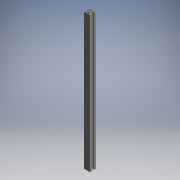
# Autodesk Inventor part: NFSF5-2020-437-Z6-YA10-YB427
Saved by Autodesk Inventor 2017.3 (Build 213256000, 256)
## iProperties
Part Number: NFSF5-2020-437-Z6-YA10-YB427
Material: Generic
Catalog Web Link: www.cadenas.de
Description: NFS5-2020, NFSB5-2020, HFS5-2020, HFSB5-2020, CAF5-2020, HFSY5-2020, NFSF5-2020, HFSF5-2020, HFSFB5-2020, NFST5-2020, HFST5-2020, HFSTB5-2020, HFSH5-2020, HFSC5-2020-HFS5 Series Aluminum Extrusions 20 Square -1 Slot-
Vendor: MISUMI
Document SubType Name: Modeling
Designer: partserver
Manufacturer: MISUMI
Mass: 84.1199 g
Surface Area: 795.09 cm^2
Volume: 84.1199 cm^3
Density: 1 g/cm^3
Appearance: PSOLRGB-175-175-175
Category: PARTsolutions
Company: MISUMI
Title: NFSF5-2020-437-Z6-YA10-YB427
Author: Cadenas PARTsolutions
Comments: HFS5 Series Aluminum Extrusions 20 Square -1 Slot-
PSOL_IDENT_0: {$CADENAS_DATA\23d-libs\misumi\metric\38_al_extrusions_blackets\5\hfs5_2020.prj},706 {VTYP=3D},{NB=N
PSOL_IDENT_1: FSF5-2020-437-Z6-YA10-YB427},{LINA=NFSF5-2020-437-Z6-YA10-YB427},{NN=NFS5-2020, NFSB5-2020, HFS5-202
PSOL_IDENT_2: 0, HFSB5-2020, CAF5-2020, HFSY5-2020, NFSF5-2020, HFSF5-2020, HFSFB5-2020, NFST5-2020, HFST5-2020, H
PSOL_IDENT_3: FSTB5-2020, HFSH5-2020, HFSC5-2020},{DATE=09.09.2019 15:28:27},{GEOMDATE=18.06.2019 07:59:14},{VERSI
PSOL_IDENT_4: ON=},{LINEID=40},{WBVAR=L,ALT1,ALT2,ALT4,ALT5,CP5,DL5,DR5,ALT6,ALT9,ALT10,ALT11,HP6,NHL6,DL6,NHR6,DR
PSOL_IDENT_5: 6,ALT7,ALT8,NH9,AH,BH,CH,DH,EH,NH10,AV,BV,CV,DV,EV,NH11,AP,BP,CP,DP,EP,ALT12,ALT13,Z,NH12,XA,XB,XC,X
PSOL_IDENT_6: D,XE,NH13,YA,YB,YC,YD,YE,ALT16,HP16,DL16,DR16,ALT17,HQ17,JLP,ALT20},{WBNUMERIC=L,NH9,AH,BH,CH,DH,EH,
PSOL_IDENT_7: NH10,AV,BV,CV,DV,EV,NH11,AP,BP,CP,DP,EP,NH12,XA,XB,XC,XD,XE,NH13,YA,YB,YC,YD,YE,HQ17,JLP}  {NB=NFSF5
PSOL_IDENT_8: -2020-437-Z6-YA10-YB427},{LINA=NFSF5-2020-437-Z6-YA10-YB427},{KT=DUMMY},{PN=NFSF5-2020-437-Z6-YA10-Y
PSOL_IDENT_9: B427},{TPS=NFSF5-2020},{MAT=6063-T5 Aluminum Alloy},{ST=Clear Anodize},{FRMW=20},{FRMH=20},{FRD=4.2}
PSOL_IDENT_10: ,{L=437},{MASS=0.53},{SA=195},{LX=0.834x10^4},{LY=0.746x10^4},{ALT1=},{M1=0},{DPL1=0},{DPR1=0},{ALT1
PSOL_IDENT_11: PN=},{ALT2=},{ALT2ALG= '','w/o End Tapping (Heli-Coil Insert)','LHP','with LHP (Tapping on the Left
PSOL_IDENT_12: (Heli-Coil Insert))','RHP','with RHP (Tapping on the Right (Heli-Coil Insert))','HPW','with HPW (Tap
PSOL_IDENT_13: ping on Both Ends (Heli-Coil Insert))' },{M2=0},{DP2=0},{ALT2PN=},{ALT4=},{ALT4ALG= '', 'w/o SC (Hig
PSOL_IDENT_14: h Precision Cut)', 'SC', 'with SC (High Precision Cut)' },{ALT4PN=},{ALT5=},{ALT5ALG= '','w/o 45 Deg
PSOL_IDENT_15: ree Cut','1','with 45 Degree Cut' },{CP5=},{CP5ALG= '','N/A' },{DL5=},{DL5ALG= '','N/A' },{DR5=},{DR
PSOL_IDENT_16: 5ALG= '','N/A' },{FRMLALT5=0},{FRMRALT5=0},{ALT5PN=},{ALT6=},{ALT6ALG= '','w/o Fastening Location Wr
PSOL_IDENT_17: ench Access Hole Alterations','1','with Fastening Location Wrench Access Hole Alterations' },{ALT9=}
PSOL_IDENT_18: ,{ALT9ALG= '','w/o Location Specified Wrench Access Hole Alteratons (Horizontal)','1','with Location
PSOL_IDENT_19: Specified Wrench Access Hole Alteratons (Horizontal)' },{ALT10=},{ALT10ALG= '','w/o Location Specif
PSOL_IDENT_20: ied Wrench Access Hole Alteratons (Vertical)','1','with Location Specified Wrench Access Hole Altera
PSOL_IDENT_21: tons (Vertical)' },{ALT11=},{ALT11ALG= '','w/o Location Specified Wrench Access Hole Alteratons (Cri
PSOL_IDENT_22: sscross)','1','with Location Specified Wrench Access Hole Alteratons (Crisscross)' },{HP6=},{HP6ALG=
PSOL_IDENT_23: '','N/A' },{NHL6=},{NHL6ALG= '','N/A' },{DL6=},{DL6ALG= '','N/A' },{NHR6=},{NHR6ALG= '','N/A' },{DR
PSOL_IDENT_24: 6=},{DR6ALG= '','N/A' },{HL6=0.000},{HL6D=0},{HR6=0.000},{HR6D=0},{J6=0},{J6D=0},{K6=0},{K6D=0},{DD6=
PSOL_IDENT_25: 0.00},{DD6ALG=0},{ALT7=},{ALT7ALG= '','N/A' },{ALT8=},{ALT8ALG= '','N/A' },{ALT678PN=},{NH9=0},{NH9M
PSOL_IDENT_26: AX=5},{NH9ALG=[0]},{AH=0.0},{AHMIN=7},{AHMAX=432},{AHALG=[0]},{BH=0.0},{BHMIN=2},{BHMAX=434},{BHALG=
PSOL_IDENT_27: [0]},{CH=0.0},{CHMIN=2},{CHMAX=436},{CHALG=[0]},{DH=0.0},{DHMIN=2},{DHMAX=438},{DHALG=[0]},{EH=0.0},
PSOL_IDENT_28: {EHMIN=2},{EHMAX=430},{EHALG=[0]},{NH10=0},{NH10MAX=5},{NH10ALG=[0]},{AV=0.0},{AVMIN=7},{AVMAX=432},
PSOL_IDENT_29: {AVALG=[0]},{BV=0.0},{BVMIN=2},{BVMAX=434},{BVALG=[0]},{CV=0.0},{CVMIN=2},{CVMAX=436},{CVALG=[0]},{D
PSOL_IDENT_30: V=0.0},{DVMIN=2},{DVMAX=438},{DVALG=[0]},{EV=0.0},{EVMIN=2},{EVMAX=430},{EVALG=[0]},{NH11=0},{NH11MA
PSOL_IDENT_31: X=5},{NH11ALG=[0]},{AP=0.0},{APMIN=7},{APMAX=432},{APALG=[0]},{BP=0.0},{BPMIN=2},{BPMAX=434},{BPALG=
PSOL_IDENT_32: [0]},{CP=0.0},{CPMIN=2},{CPMAX=436},{CPALG=[0]},{DP=0.0},{DPMIN=2},{DPMAX=438},{DPALG=[0]},{EP=0.0},
PSOL_IDENT_33: {EPMIN=2},{EPMAX=430},{EPALG=[0]},{ALT9PN=},{ALT10PN=},{ALT11PN=},{ALT91011PN=},{ALT12=},{ALT12ALG= ''
PSOL_IDENT_34: ,'w/o Counterbore Hole in Specified Position (Vertical)','1','with Counterbore Hole in Specified Pos
PSOL_IDENT_35: ition (Vertical)' },{ALT13=1},{ALT13ALG= '','w/o Counterbore Hole in Specified Position (Horizontal)'
PSOL_IDENT_36: ,'1','with Counterbore Hole in Specified Position (Horizontal)' },{Z=6},{ZALG='5','5','6','6'},{DD12=
PSOL_IDENT_37: 6.5},{DD112=11.0},{NH12=0},{NH12MAX=5},{NH12ALG=[0]},{XA=0.0},{XAMIN=7},{XAMAX=443},{XAALG=[0]},{XB=
PSOL_IDENT_38: 0.0},{XBMIN=13},{XBMAX=456},{XBALG=[0]},{XC=0.0},{XCMIN=13},{XCMAX=469},{XCALG=[0]},{XD=0.0},{XDMIN=
PSOL_IDENT_39: 13},{XDMAX=482},{XDALG=[0]},{XE=0.0},{XEMIN=13},{XEMAX=430},{XEALG=[0]},{NH13=2},{NH13MAX=5},{NH13AL
PSOL_IDENT_40: G=[1:5/1]},{YA=10.0},{YAMIN=7},{YAMAX=417},{YAALG=[7:417/0.5]},{YB=427.0},{YBMIN=23},{YBMAX=430},{YB
PSOL_IDENT_41: ALG=[23:430/0.5]},{YC=0.0},{YCMIN=440},{YCMAX=443},{YCALG=[0]},{YD=0.0},{YDMIN=13},{YDMAX=456},{YDAL
PSOL_IDENT_42: G=[0]},{YE=0.0},{YEMIN=13},{YEMAX=430},{YEALG=[0]},{ALT12PN=},{ALT13PN=-YA10-YB427},{ALT1213PN=-Z6-Y
PSOL_IDENT_43: A10-YB427},{ALT16=},{ALT16ALG= '','w/o M Type Hole Alteration','1','with M Type Hole Alteration' },{
PSOL_IDENT_44: HP16=},{HP16ALG= '','N/A' },{DL16=},{DL16ALG= '','N/A' },{DR16=},{DR16ALG= '','N/A' },{H116=0},{D16=
PSOL_IDENT_45: 0.0},{ALT16PN=},{ALT17=},{ALT17ALG= '','w/o L Type Hole Alteration (Top)','1','with L Type Hole Alte
PSOL_IDENT_46: ration (Top)' },{HQ17=0},{HQ17ALG=0},{JLP=0},{JLPMIN=4.9},{JLPMAX=0},{JLPALG=[0]},{L17=0},{D17=0.0},
PSOL_IDENT_47: {ALT17PN=},{ALT20=},{ALT20PN=},{ERRORALT01=OK},{ERRORALT02=OK},{ERRORALT05=OK},{ERRORALT06091=OK},{E
PSOL_IDENT_48: RRORALT06092=OK},{ERRORALT06093=OK},{ERRORALT06094=OK},{ERRORALT06101=OK},{ERRORALT06102=OK},{ERRORA
PSOL_IDENT_49: LT06103=OK},{ERRORALT06104=OK},{ERRORALT06111=OK},{ERRORALT06112=OK},{ERRORALT06113=OK},{ERRORALT061
PSOL_IDENT_50: 14=OK},{ERRORALT06121=OK},{ERRORALT06122=OK},{ERRORALT06123=OK},{ERRORALT06124=OK},{ERRORALT06131=OK
PSOL_IDENT_51: },{ERRORALT06132=OK},{ERRORALT06133=OK},{ERRORALT06134=OK},{ERRORALT0616=OK},{ERRORALT06171=OK},{ERR
PSOL_IDENT_52: ORALT06172=OK},{ERRORALT06173=OK},{ERRORALT0911=OK},{ERRORALT0913=OK},{ERRORALT0916=OK},{ERRORALT091
PSOL_IDENT_53: 7=OK},{ERRORALT1011=OK},{ERRORALT1012=OK},{ERRORALT1016=OK},{ERRORALT1017=OK},{ERRORALT1112=OK},{ERR
PSOL_IDENT_54: ORALT1113=OK},{ERRORALT1116=OK},{ERRORALT1117=OK},{ERRORALT1216=OK},{ERRORALT1217=OK},{ERRORALT1316=
PSOL_IDENT_55: OK},{ERRORALT1317=OK},{ERRORALT1617=OK},{ERRORPN=},{TFW=0}
NB: NFSF5-2020-437-Z6-YA10-YB427
NN: NFS5-2020, NFSB5-2020, HFS5-2020, HFSB5-2020, CAF5-2020, HFSY5-2020, NFSF5-2020, HFSF5-2020, HFSFB5-2020, NFST5-2020, HFST5-2020, HFSTB5-2020, HFSH5-2020, HFSC5-2020
NT: HFS5 Series Aluminum Extrusions 20 Square -1 Slot-
NBSYN: $PN.
LINA: NFSF5-2020-437-Z6-YA10-YB427
CATALOG: Misumi
PN: NFSF5-2020-437-Z6-YA10-YB427
TPS: NFSF5-2020
MAT: 6063-T5 Aluminum Alloy
ST: Clear Anodize
L: 437
MASS: 0.53
SA: 195
LX: 0.834x10^4
LY: 0.746x10^4
ALT1: w/o End Tapping
M1: 0
DPL1: 0
DPR1: 0
ALT2: w/o End Tapping (Heli-Coil Insert)
M2: 0
DP2: 0
ALT4: w/o SC (High Precision Cut)
ALT5: w/o 45 Degree Cut
CP5: N/A
DL5: N/A
DR5: N/A
ALT6: w/o Fastening Location Wrench Access Hole Alterations
ALT9: w/o Location Specified Wrench Access Hole Alteratons (Horizontal)
ALT10: w/o Location Specified Wrench Access Hole Alteratons (Vertical)
ALT11: w/o Location Specified Wrench Access Hole Alteratons (Crisscross)
HP6: N/A
NHL6: N/A
DL6: N/A
NHR6: N/A
DR6: N/A
HL6D: 0
HR6D: 0
J6D: 0
K6D: 0
DD6: 0
ALT7: N/A
ALT8: N/A
NH9: 0
AH: 0
BH: 0
CH: 0
DH: 0
EH: 0
NH10: 0
AV: 0
BV: 0
CV: 0
DV: 0
EV: 0
NH11: 0
AP: 0
BP: 0
CP: 0
DP: 0
EP: 0
ALT12: w/o Counterbore Hole in Specified Position (Vertical)
ALT13: with Counterbore Hole in Specified Position (Horizontal)
Z: 6
DD12: 6.5
DD112: 11
NH12: 0
XA: 0
XB: 0
XC: 0
XD: 0
XE: 0
NH13: 2
YA: 10
YB: 427
YC: 0
YD: 0
YE: 0
ALT16: w/o M Type Hole Alteration
HP16: N/A
DL16: N/A
DR16: N/A
H116: 0
D16: 0
ALT17: w/o L Type Hole Alteration (Top)
HQ17: 0
JLP: 0
D17: 0
ALT20: w/o CW (End Face C Chamfering)
SUPPLIER: MISUMI
ARTICLENO: NFSF5-2020-437-Z6-YA10-YB427
BOMINFO: NFSF5-2020-437-Z6-YA10-YB427
CREATOR: CADENAS GmbH
Autodesk Inventor part; units mm, degrees
ref_plane "YZ Plane" through (0, 0, 0) normal (1, 0, 0) x (0, 1, 0)
ref_plane "XZ Plane" through (0, 0, 0) normal (0, 1, 0) x (-1, 0, 0)
ref_plane "XY Plane" through (0, 0, 0) normal (0, 0, 1) x (1, 0, 0)
sketch "Sketch_76" plane through (0, 0, 0) normal (0, 0, 1) x (1, 0, 0)
  line L0 (-10, -3) -> (-10, -9)
  arc A0 (-10, -9) -> (-9, -10) centre (-9, -9) ccw
  line L1 (-9, -10) -> (9, -10)
  arc A1 (9, -10) -> (10, -9) centre (9, -9) ccw
  line L2 (10, -9) -> (10, -3)
  line L3 (10, -3) -> (8, -3)
  line L4 (8, -3) -> (8, -6)
  line L5 (8, -6) -> (7.0607, -6)
  line L6 (7.0607, -6) -> (4, -2.9393)
  line L7 (4, -2.9393) -> (4, -0.6536)
  arc A2 (4, -0.6536) -> (3.933, -0.4036) centre (3.5, -0.6536) ccw
  line L8 (3.933, -0.4036) -> (3.7, 0)
  line L9 (3.7, 0) -> (3.933, 0.4036)
  arc A3 (3.933, 0.4036) -> (3.933, 0.9036) centre (3.5, 0.6536) ccw
  line L10 (3.933, 0.9036) -> (3.751, 1.2189)
  line L11 (3.751, 1.2189) -> (4, 2.5)
  line L12 (4, 2.5) -> (4, 2.9393)
  line L13 (4, 2.9393) -> (7.0607, 6)
  line L14 (7.0607, 6) -> (8, 6)
  line L15 (8, 6) -> (8, 3)
  line L16 (8, 3) -> (10, 3)
  line L17 (10, 3) -> (10, 9)
  arc A4 (10, 9) -> (9, 10) centre (9, 9) ccw
  line L18 (9, 10) -> (3, 10)
  line L19 (3, 10) -> (3, 8)
  line L20 (3, 8) -> (6, 8)
  line L21 (6, 8) -> (6, 7.0607)
  line L22 (6, 7.0607) -> (2.9393, 4)
  line L23 (2.9393, 4) -> (0.6536, 4)
  arc A5 (0.6536, 4) -> (0.4036, 3.933) centre (0.6536, 3.5) ccw
  line L24 (0.4036, 3.933) -> (0, 3.7)
  line L25 (0, 3.7) -> (-0.4036, 3.933)
  arc A6 (-0.4036, 3.933) -> (-0.9036, 3.933) centre (-0.6536, 3.5) ccw
  line L26 (-0.9036, 3.933) -> (-1.2189, 3.751)
  line L27 (-1.2189, 3.751) -> (-2.5, 4)
  line L28 (-2.5, 4) -> (-2.9393, 4)
  line L29 (-2.9393, 4) -> (-6, 7.0607)
  line L30 (-6, 7.0607) -> (-6, 8)
  line L31 (-6, 8) -> (-3, 8)
  line L32 (-3, 8) -> (-3, 10)
  line L33 (-3, 10) -> (-9, 10)
  arc A7 (-9, 10) -> (-10, 9) centre (-9, 9) ccw
  line L34 (-10, 9) -> (-10, 3)
  line L35 (-10, 3) -> (-8, 3)
  line L36 (-8, 3) -> (-8, 6)
  line L37 (-8, 6) -> (-7.0607, 6)
  line L38 (-7.0607, 6) -> (-4, 2.9393)
  line L39 (-4, 2.9393) -> (-4, 0.6536)
  arc A8 (-4, 0.6536) -> (-3.933, 0.4036) centre (-3.5, 0.6536) ccw
  line L40 (-3.933, 0.4036) -> (-3.7, 0)
  line L41 (-3.7, 0) -> (-3.933, -0.4036)
  arc A9 (-3.933, -0.4036) -> (-3.933, -0.9036) centre (-3.5, -0.6536) ccw
  line L42 (-3.933, -0.9036) -> (-3.751, -1.2189)
  line L43 (-3.751, -1.2189) -> (-4, -2.5)
  line L44 (-4, -2.5) -> (-4, -2.9393)
  line L45 (-4, -2.9393) -> (-7.0607, -6)
  line L46 (-7.0607, -6) -> (-8, -6)
  line L47 (-8, -6) -> (-8, -3)
  line L48 (-8, -3) -> (-10, -3)
  line L49 (-6, -7.2678) -> (-6, -7.5)
  arc A10 (-6, -7.5) -> (-5.5, -8) centre (-5.5, -7.5) ccw
  line L50 (-5.5, -8) -> (5.5, -8)
  arc A11 (5.5, -8) -> (6, -7.5) centre (5.5, -7.5) ccw
  line L51 (6, -7.5) -> (6, -7.2678)
  arc A12 (6, -7.2678) -> (5.8536, -6.9142) centre (5.5, -7.2678) ccw
  line L52 (5.8536, -6.9142) -> (3.0858, -4.1464)
  arc A13 (3.0858, -4.1464) -> (2.7322, -4) centre (2.7322, -4.5) ccw
  line L53 (2.7322, -4) -> (-2.7322, -4)
  arc A14 (-2.7322, -4) -> (-3.0858, -4.1464) centre (-2.7322, -4.5) ccw
  line L54 (-3.0858, -4.1464) -> (-5.8536, -6.9142)
  arc A15 (-5.8536, -6.9142) -> (-6, -7.2678) centre (-5.5, -7.2678) ccw
  constraints: 110 end point, 32 point on circle, 16 centre point
extrude "Extrusion1" add sketch "Sketch_76" against normal blind 437
sketch "Sketch2" plane through (0, 0, -437) normal (0, 0, -1) x (-1, 0, 0)
  point P0 (0, 0)
hole "Hole1" at (0, 0, -437) direction (0, 0, 1) diameter 4.2 depth 437
sketch "Sketch_50" plane through (0, 0, 0) normal (0, 1, 0) x (1, 0, 0)
  line L0 (10, 10) -> (-10, 10)
  line L1 (-10, 10) -> (-10, 13.25)
  line L2 (-10, 13.25) -> (4, 13.25)
  line L3 (4, 13.25) -> (4, 15.5)
  line L4 (4, 15.5) -> (10, 15.5)
  line L5 (10, 15.5) -> (10, 10)
  line L6 (10, 10) -> (-10, 10)
  constraints: 14 end point
revolve "Revolution1" cut sketch "Sketch_50" angle 360 about axis through (10, 0, -10) along (1, 0, 0)
sketch "Sketch_51" plane through (0, 0, 0) normal (0, 1, 0) x (1, 0, 0)
  line L0 (10, 427) -> (-10, 427)
  line L1 (-10, 427) -> (-10, 430.25)
  line L2 (-10, 430.25) -> (4, 430.25)
  line L3 (4, 430.25) -> (4, 432.5)
  line L4 (4, 432.5) -> (10, 432.5)
  line L5 (10, 432.5) -> (10, 427)
  line L6 (10, 427) -> (-10, 427)
  constraints: 14 end point
revolve "Revolution2" cut sketch "Sketch_51" angle 360 about axis through (10, 0, -427) along (1, 0, 0)
ref_plane "C1_XY" through (0, 0, 0) normal (0, 0, 1) x (1, 0, 0)
ref_plane "C1_YZ" through (0, 0, 0) normal (1, 0, 0) x (0, 1, 0)
ref_plane "C1_ZX" through (0, 0, 0) normal (0, 1, 0) x (0, 0, 1)
body "Solid1"
